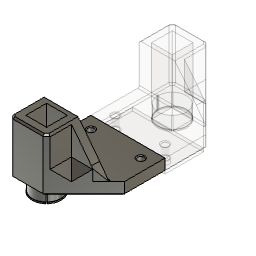
Stützenklemme vorne v5 (Autodesk Fusion 360 design; units mm, degrees)
Autodesk Fusion 360 part; units mm, degrees
note: some values were not read from the file. Set by a fixed rule: which sketch regions a step uses.
sketch "Skizze1" plane through (0, 0, 0) normal (0, 0, 1) x (1, 0, 0)
  line L0 (-50, 0) -> (-91.23, 0)
  line L1 (-91.23, 0) -> (-91.23, 100)
  line L2 (-91.23, 100) -> (0, 100)
  line L3 (0, 100) -> (0, 50)
  line L4 (0, 50) -> (-50, 0)
  dimension "d1" = 91.23
  dimension "d2" = 100
  dimension "d3" = 41.23
  dimension "d4" = 50
  dimension "d5" = 50
  dimension "d6" = 50
  constraint horizontal L0
  constraint perpendicular L0 L1
  constraint perpendicular L1 L2
  constraint perpendicular L2 L3
  measures "d1" distance of L1.end L2.end
  measures "d2" distance of L0.end L1.end
  measures "d3" distance of L0.end L0.start
  measures "d4" distance of L2.end L3.end
  measures "d5" distance of origin L0.start
  measures "d6" distance of origin L3.end
extrude "Extrusion1" add sketch "Skizze1" along normal blind 15 makes body 1
sketch "Skizze2" plane through (0, 0, 15) normal (0, 0, 1) x (-1, 0, 0)
  line L0 (0, -50) -> (0, -100)
  line L1 (0, -100) -> (91.23, -100)
  line L2 (91.23, -100) -> (91.23, 0)
  line L3 (91.23, 0) -> (50, 0)
  line L4 (50, 0) -> (0, -50)
  line L5 (81.23, -10) -> (55.73, -10)
  line L6 (55.73, -10) -> (55.73, -35.5)
  line L7 (55.73, -35.5) -> (81.23, -35.5)
  line L8 (81.23, -35.5) -> (81.23, -10)
  line L9 (91.23, -40.5) -> (9.5, -40.5)
  line L10 (45.73, -40.5) -> (45.73, 0)
  dimension "d9" = 25.5
  dimension "d10" = 25.5
  dimension "d11" = 10
  dimension "d12" = 10
  dimension "d13" = 5
  dimension "d14" = 10
  constraint horizontal L5
  constraint vertical L6
  constraint horizontal L7
  constraint vertical L8
  constraint coincident L2 L9.start
  constraint coincident L4 L9.end
  constraint perpendicular L2 L9
  constraint coincident L9 L10.start
  constraint coincident L3 L10.end
  constraint perpendicular L3 L10
  measures "d9" distance of L6.end L7.end
  measures "d10" distance of L5.start L7.end
  measures "d11" distance of L2 L8
  measures "d12" distance of L3 L5
  measures "d13" distance of L7 L9
  measures "d14" distance of L6 L10
extrude "Extrusion2" add sketch "Skizze2" along normal blind 50 contours L2 L3 L4 L9 L10 bodies 1
chamfer "Fase2" distance 4 angle 45 1 edges at (-91.23, 0, 32.5) on bodies 1
sketch "Skizze4" plane through (0, 0, 15) normal (0, 0, 1) x (-1, 0, 0)
  line L0 (45.73, -40.5) -> (45.73, -4.27)
  line L1 (45.73, -4.27) -> (0, -50)
  line L2 (0, -50) -> (0, -100)
  line L3 (0, -100) -> (91.23, -100)
  line L4 (91.23, -100) -> (91.23, -40.5)
  line L5 (91.23, -40.5) -> (45.73, -40.5)
  line L6 (45.73, -40.5) -> (9.5, -40.5)
  line L7 (9.5, -40.5) -> (19.5, -30.5)
  line L8 (45.73, -30.5) -> (45.73, -40.5)
  line L9 (45.73, -30.5) -> (19.5, -30.5)
  dimension "d23" = 10
  constraint coincident L0.start L5.end
  constraint coincident L1 L6.end
  constraint perpendicular L0 L6
  constraint coincident L1 L7.end
  constraint parallel L1 L7
  constraint coincident L0 L8.start
  constraint perpendicular L6 L8
  measures "d23" distance of L6 L9
extrude "Extrusion3" add sketch "Skizze4" along normal blind 50 contours L0 L1 L6 L7 L8 L9 bodies 1
sketch "Skizze6" plane through (0, 40.5, 0) normal (0, 1, 0) x (-1, 0, 0)
  line L0 (9.5, 15) -> (91.23, 15)
  line L1 (91.23, 15) -> (91.23, 65)
  line L2 (91.23, 65) -> (9.5, 65)
  line L3 (9.5, 65) -> (9.5, 15)
  line L4 (9.5, 15) -> (45.93, 65)
  line L5 (45.93, 15) -> (9.5, 15)
  line L6 (45.93, 65) -> (45.93, 15)
  dimension "d26" = 45.3
  constraint coincident L0.start L3.end
  constraint coincident L2 L4.end
  constraint coincident L0 L5.start
  constraint perpendicular L0 L6
  measures "d26" distance of L1 L6
extrude "Extrusion4" cut sketch "Skizze6" against normal blind 20 contours L2 L3 L4 bodies 1
chamfer "Fase5" distance 13 angle 45 2 edges at (-45.73, 17.385, 15) (-32.615, 30.5, 15) on bodies 1
extrude "Extrusion5" cut 1 faces at (-64.23, 27, 15) along direction (0, 0, -1) blind 15 on bodies 1 bodies 1
chamfer "Fase7" distance 2 angle 45 5 edges at (-91.23, 22.25, 65) (-89.23, 2, 65) (-68.615, 0, 65) (-47.865, 2.135, 65) (-45.73, 12.385, 65) on bodies 1
sketch "Skizze7" plane through (0, 30.5, 0) normal (0, -1, 0) x (1, 0, 0)
  line L0 (-45.73, 28) -> (-19.5, 28)
  line L1 (-19.5, 28) -> (-19.5, 28.725)
  line L2 (-19.5, 28.725) -> (-45.93, 65)
  line L3 (-45.93, 65) -> (-47.73, 65)
  line L4 (-47.73, 65) -> (-45.73, 63)
  line L5 (-45.73, 63) -> (-45.73, 28)
  line L6 (-47.73, 65) -> (-41.0977, 58.3677)
  constraint coincident L3.end L4.start
  constraint coincident L2 L6.end
  constraint parallel L4 L6
extrude "Extrusion6" cut sketch "Skizze7" against normal blind 32 contours L2 L3 L4 L6 bodies 1
fillet "Abrundung1" radius 642.5 1 edges at (-41.0977, 35.5, 58.3677) on bodies 1
sketch "Skizze8" plane through (0, 0, 15) normal (0, 0, 1) x (-1, 0, 0)
  line L0 (91.23, -40.5) -> (9.5, -40.5)
  line L1 (9.5, -40.5) -> (0, -50)
  line L2 (0, -50) -> (0, -100)
  line L3 (0, -100) -> (91.23, -100)
  line L4 (91.23, -100) -> (91.23, -40.5)
  circle A0 centre (76.23, -85) radius 4
  circle A1 centre (15, -85) radius 4
  dimension "d39" = 15
  dimension "d40" = 8
  dimension "d41" = 15
  dimension "d42" = 15
  constraint equal A0 A1
  constraint horizontal A0.centre A1.centre
  measures "d39" distance of L3 A0.centre
  measures "d40" diameter of A0
  measures "d41" distance of L4 A0.centre
  measures "d42" distance of L2 A1.centre
fillet "Abrundung2" radius 2 1 edges at (-50.365, 40.5, 15) on bodies 1
extrude "Extrusion7" cut sketch "Skizze8" against normal blind 15 contours A0 | A1 bodies 1
sketch "Skizze9" plane through (0, 0, 0) normal (0, 0, -1) x (1, 0, 0)
  circle A0 centre (-15, -85) radius 4
  circle A1 centre (-76.23, -85) radius 4
  line L0 (-55.73, -10) -> (-55.73, -35.5)
  line L1 (-55.73, -35.5) -> (-81.23, -35.5)
  line L2 (-81.23, -35.5) -> (-81.23, -10)
  line L3 (-81.23, -10) -> (-55.73, -10)
  line L4 (-87.23, 0) -> (-91.23, -4)
  line L5 (-91.23, -4) -> (-91.23, -100)
  line L6 (-91.23, -100) -> (0, -100)
  line L7 (0, -100) -> (0, -50)
  line L8 (0, -50) -> (-50, 0)
  line L9 (-50, 0) -> (-87.23, 0)
  line L10 (-81.23, -10) -> (-55.73, -35.5) construction
  line L11 (-55.73, -10) -> (-81.23, -35.5) construction
  circle A2 centre (-68.48, -22.75) radius 17.45
  dimension "d47" = 34.9
  constraint coincident L2.end L3.start
  constraint coincident L0.end L1.start
  constraint coincident L0.start L3.end
  constraint coincident L1.end L2.start
  constraint midpoint L11 A2.centre
  measures "d47" diameter of A2
extrude "Extrusion8" add sketch "Skizze9" along normal blind 15 contours L0 A2 | L3 A2 | L1 A2 | L2 A2 bodies 1
sketch "Skizze10" plane through (0, 0, -15) normal (0, 0, -1) x (1, 0, 0)
  line L0 (-80.3939, -10) -> (-56.5661, -10)
  arc A0 (-56.5661, -10) -> (-80.3939, -10) centre (-68.48, -22.75) ccw
  arc A1 (-56.2248, -9.6347) -> (-80.7352, -9.6347) centre (-68.48, -22.75) ccw
  line L1 (-80.7352, -9.6347) -> (-80.3939, -10)
  line L2 (-56.5661, -10) -> (-56.2248, -9.6347)
  dimension "d50" = 0.5
  constraint coincident L0.start A0.end
  constraint coincident L0.end A0.start
sketch "Skizze11" plane through (0, 0, -15) normal (0, 0, -1) x (1, 0, 0)
  arc A0 (-55.73, -34.6639) -> (-55.73, -10.8361) centre (-68.48, -22.75) ccw
  line L0 (-55.73, -10.8361) -> (-55.73, -34.6639)
  arc A1 (-55.3647, -35.0052) -> (-55.3647, -10.4948) centre (-68.48, -22.75) ccw
  line L1 (-55.73, -10.8361) -> (-55.3647, -10.4948)
  line L2 (-55.3647, -35.0052) -> (-55.73, -34.6639)
  dimension "d51" = 0.5
  constraint coincident A0.end L0.start
  constraint coincident A0.start L0.end
sketch "Skizze12" plane through (0, 0, -15) normal (0, 0, -1) x (1, 0, 0)
  line L0 (-56.5661, -35.5) -> (-80.3939, -35.5)
  arc A0 (-80.3939, -35.5) -> (-56.5661, -35.5) centre (-68.48, -22.75) ccw
  arc A1 (-80.7352, -35.8653) -> (-56.2248, -35.8653) centre (-68.48, -22.75) ccw
  line L1 (-80.7352, -35.8653) -> (-80.3939, -35.5)
  line L2 (-56.2248, -35.8653) -> (-56.5661, -35.5)
  dimension "d52" = 0.5
  constraint coincident L0.end A0.start
  constraint coincident L0.start A0.end
sketch "Skizze13" plane through (0, 0, -15) normal (0, 0, -1) x (1, 0, 0)
  line L0 (-81.23, -34.6639) -> (-81.23, -10.8361)
  arc A0 (-81.23, -10.8361) -> (-81.23, -34.6639) centre (-68.48, -22.75) ccw
  arc A1 (-81.5953, -10.4948) -> (-81.5953, -35.0052) centre (-68.48, -22.75) ccw
  line L1 (-81.23, -10.8361) -> (-81.5953, -10.4948)
  line L2 (-81.5953, -35.0052) -> (-81.23, -34.6639)
  dimension "d53" = 0.5
  constraint coincident L0.end A0.start
  constraint coincident L0.start A0.end
extrude "Extrusion9" add sketch "Skizze11" sketch "Skizze13" sketch "Skizze10" sketch "Skizze12" along normal blind 1.5 of sketch 2 of sketch 3 of sketch 4 bodies 1
chamfer "Fase9" distance 2 angle 45 6 edges at (-68.615, 0, 0) (-25, 25, 0) (0, 75, 0) (-45.615, 100, 0) (-91.23, 52, 0) (-89.23, 2, 0) on bodies 1
sketch "Skizze14" plane through (0, 0, 0) normal (0, 0, -1) x (1, 0, 0)
  circle A0 centre (-15, -85) radius 4
  circle A1 centre (-76.23, -85) radius 4
  arc A2 (-81.23, -10.8361) -> (-81.23, -34.6639) centre (-68.48, -22.75) ccw
  line L0 (-81.23, -10.8361) -> (-81.23, -10)
  line L1 (-81.23, -10) -> (-80.3939, -10)
  arc A3 (-56.5661, -10) -> (-80.3939, -10) centre (-68.48, -22.75) ccw
  line L2 (-56.5661, -10) -> (-55.73, -10)
  line L3 (-55.73, -10) -> (-55.73, -10.8361)
  arc A4 (-55.73, -34.6639) -> (-55.73, -10.8361) centre (-68.48, -22.75) ccw
  line L4 (-55.73, -34.6639) -> (-55.73, -35.5)
  line L5 (-55.73, -35.5) -> (-56.5661, -35.5)
  arc A5 (-80.3939, -35.5) -> (-56.5661, -35.5) centre (-68.48, -22.75) ccw
  line L6 (-80.3939, -35.5) -> (-81.23, -35.5)
  line L7 (-81.23, -35.5) -> (-81.23, -34.6639)
  line L8 (-89.23, -98) -> (-2, -98)
  line L9 (-2, -98) -> (-2, -50.8284)
  line L10 (-2, -50.8284) -> (-50.8284, -2)
  line L11 (-50.8284, -2) -> (-86.4016, -2)
  line L12 (-86.4016, -2) -> (-89.23, -4.8284)
  line L13 (-89.23, -4.8284) -> (-89.23, -98)
  line L14 (-85.9139, -22) -> (-86.7255, -22)
  line L15 (-86.7255, -23.5) -> (-85.9139, -23.5)
  line L16 (-81.23, -10.8361) -> (-89.23, -10.8361)
  line L17 (-81.23, -34.6639) -> (-89.23, -34.6639)
  line L18 (-89.23, -22.75) -> (-78, -22.75) construction
  line L19 (-86.7255, -22) -> (-86.7255, -23.5)
  dimension "d57" = 11.9139
  dimension "d58" = 23.8277
  dimension "d59" = 1.5
  constraint perpendicular L13 L14
  constraint coincident A2 L15.end
  constraint perpendicular L13 L15
  constraint coincident A2.start L0.start
  constraint coincident L13 L16.end
  constraint perpendicular L13 L16
  constraint coincident A2.end L7.end
  constraint coincident L13 L17.end
  constraint perpendicular L13 L17
  constraint coincident L13 L18.start
  constraint symmetric L14.end L15.start L18
  constraint perpendicular L14 L19
  constraint coincident A2 L14.start
  measures "d57" distance of L16.end L18.start
  measures "d58" distance of L16.end L17.end
  measures "d59" distance of L14.end L15.start
extrude "Extrusion10" add sketch "Skizze14" along normal blind 15 contours A2 L14 L15 L19 bodies 1
extrude "Extrusion11" add 1 faces at (-86.6264, 22.8334, -15) along direction (0, 0, -1) blind 1.5 on bodies 1 bodies 1
mirror "Spiegeln1" about plane through (-91.23, 100, 0) normal (0, 1, 0) of bodies 1 makes body 2
chamfer "Fase10" distance 1 angle 45 2 edges at (-11.2707, 83.5535, 15) (-72.5007, 83.5535, 15) on bodies 1
chamfer "Fase11" distance 1 angle 45 2 edges at (-11.2707, 116.4465, 15) (-72.5007, 116.4465, 15) on bodies 2
sketch "Skizze1 (2)" plane through (0, 0, 0) normal (0, 0, -1) x (1, 0, 0) in component "ReparaturPlatte"
  line L0 (-2, -102) -> (-89.23, -102)
  line L1 (-89.23, -102) -> (-89.23, -195.1716)
  line L2 (-89.23, -195.1716) -> (-86.4016, -198)
  line L3 (-86.4016, -198) -> (-50.8284, -198)
  line L4 (-50.8284, -198) -> (-2, -149.1716)
  line L5 (-2, -149.1716) -> (-2, -102)
  line L6 (-86.7255, -176.5) -> (-85.9139, -176.5)
  arc A0 (-81.23, -165.3361) -> (-85.9139, -176.5) centre (-68.48, -177.25) ccw
  line L7 (-81.23, -165.3361) -> (-81.23, -164.5)
  line L8 (-81.23, -164.5) -> (-80.3939, -164.5)
  arc A1 (-56.5661, -164.5) -> (-80.3939, -164.5) centre (-68.48, -177.25) ccw
  line L9 (-56.5661, -164.5) -> (-55.73, -164.5)
  line L10 (-55.73, -164.5) -> (-55.73, -165.3361)
  arc A2 (-55.73, -189.1639) -> (-55.73, -165.3361) centre (-68.48, -177.25) ccw
  line L11 (-55.73, -189.1639) -> (-55.73, -190)
  line L12 (-55.73, -190) -> (-56.5661, -190)
  arc A3 (-80.3939, -190) -> (-56.5661, -190) centre (-68.48, -177.25) ccw
  line L13 (-80.3939, -190) -> (-81.23, -190)
  line L14 (-81.23, -190) -> (-81.23, -189.1639)
  arc A4 (-85.9139, -178) -> (-81.23, -189.1639) centre (-68.48, -177.25) ccw
  line L15 (-85.9139, -178) -> (-86.7255, -178)
  line L16 (-86.7255, -178) -> (-86.7255, -176.5)
  circle A5 centre (-76.23, -115) radius 4
  circle A6 centre (-15, -115) radius 4
  line L17 (-89.23, -102) -> (-2, -102)
  line L18 (-2, -102) -> (-2, -149.1716)
  line L19 (-2, -149.1716) -> (-89.23, -149.1716)
  line L20 (-89.23, -149.1716) -> (-89.23, -102)
  circle A7 centre (-76.23, -115) radius 5.014
  circle A8 centre (-15, -115) radius 4.9973
  constraint horizontal L17
  constraint vertical L18
  constraint horizontal L19
  constraint vertical L20
  constraint coincident L4.end L5.start
  constraint coincident L0.end L1.start
  constraint concentric A5 A7
  constraint concentric A6 A8
extrude "Extrusion1'" add sketch "Skizze1 (2)" along normal blind 4 separate body contours L0 L1 L5 L17 L18 L19 L20 makes body 3 in component "ReparaturPlatte"
copy_body "Körper->Berechn1" bodies 1 removing the originals makes body 4 in component "Component'"
component "ReparaturPlatte" placed x (1, 0, 0) y (0, 1, 0) z (0, 0, 1) at (0, 0, 0)
component "Component'" placed x (1, 0, 0) y (0, 1, 0) z (0, 0, 1) at (0, 0, 0)
equation "d1 = 100.00 mm - 8.77 mm"
equation "d3 = 50.00 mm - 8.77 mm"
equation "d57 = d58 / 2"
